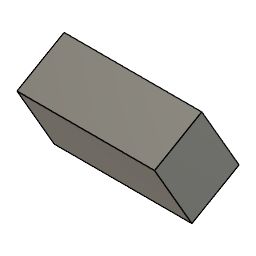
replay (Autodesk Fusion 360 design; units mm, degrees)
Autodesk Fusion 360 part; units mm, degrees
ref_plane "工作平面1" through (12.125, 0, 0) normal (0, 0.866025, 0.5) x (1, 0, 0)
sketch "草图1" plane through (0, 0, 0) normal (0, 0.866025, 0.5) x (1, 0, 0)
  line L0 (48, -19) -> (48, 0)
  line L1 (48, 0) -> (0, 0)
  line L2 (0, 0) -> (0, -19)
  line L3 (0, -19) -> (48, -19)
extrude "拉伸1" add sketch "草图1" along normal blind 26
